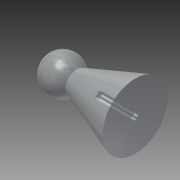
# Autodesk Inventor part: pion
Saved by Autodesk Inventor 2015 (Build 190159000, 159)
## iProperties
Created: 2015-02-16
Part Number: pion
Material: Verre
Document SubType Name: Modeling
Designer: informatique
Density: 2.18 g/cm^3
Appearance: Clair
Author: informatique
Autodesk Inventor part; units mm, degrees
ref_plane "YZ Plane" through (0, 0, 0) normal (1, 0, 0) x (0, 1, 0)
ref_plane "XZ Plane" through (0, 0, 0) normal (0, 1, 0) x (-1, 0, 0)
ref_plane "XY Plane" through (0, 0, 0) normal (0, 0, 1) x (1, 0, 0)
sketch "Esquisse1" plane through (0, 0, 0) normal (0, 1, 0) x (-1, 0, 0)
  line L0 (0, 0) -> (25, 0)
  line L1 (25, 0) -> (0, 0)
  line L2 (0, 0) -> (0, 9)
  line L3 (0, 9) -> (25, 0)
  arc A0 (25, 0) -> (15, 0) centre (20, 0) ccw
  dimension "d0" = 9
  dimension "d1" = 25
  dimension "d2" = 5
  constraints: 8 end point, 2 point on circle, 2 point on line, 1 centre point, 1 collinear, 1 horizontal, 1 vertical
  measures "d0" distance of L0.start L2.end
  measures "d1" distance of L0.start L0.end
  measures "d2" distance of L0.end A0.centre
revolve "Révolution1" add sketch "Esquisse1" angle 360 about axis through (-25, 0, 0) along (1, 0, 0)
sketch "Esquisse2" plane through (0, 0, 0) normal (1, 0, 0) x (0, 0, -1)
  line L0 (-0.3714, 0.9357) -> (0.3286, 0.9357)
  line L1 (0.3286, 0.9357) -> (0.3286, -0.9643)
  line L2 (0.3286, -0.9643) -> (-0.3714, -0.9643)
  line L3 (-0.3714, -0.9643) -> (-0.3714, 0.9357)
  line L4 (0.9286, 0.3357) -> (-0.9714, 0.3357)
  line L5 (-0.9714, 0.3357) -> (-0.9714, -0.3643)
  line L6 (-0.9714, -0.3643) -> (0.9286, -0.3643)
  line L7 (0.9286, -0.3643) -> (0.9286, 0.3357)
  point P0 (0, 0)
  dimension "d4" = 0.7
  dimension "d5" = 0.7
  dimension "d6" = 1.9
  dimension "d7" = 1.9
  dimension "d8" = 0.6
  dimension "d9" = 0.6
  constraints: 16 end point, 4 parallel, 2 horizontal, 2 perpendicular
  measures "d4" distance of L0.start L0.end
  measures "d5" distance of L6.end L4.start
  measures "d6" distance of L5.end L6.end
  measures "d7" distance of L2.end L0.start
  measures "d8" distance between parallel lines of L6 L2
  measures "d9" distance between parallel lines of L3 L5
extrude "Extrusion1" cut sketch "Esquisse2" against normal blind 10
